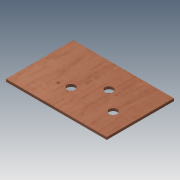
# Autodesk Inventor part: gabarito-porta-cabos
Saved by Autodesk Inventor 2017 (Build 210142000, 142)
## iProperties
Created: 2018-08-29
Part Number: gabarito-porta-cabos
Material: Wood (Oak)
Document SubType Name: Sheet Metal
Designer: Luiz Gustavo
Density: 0.76 g/cm^3
Sheet Metal Rule: Default_mm
Appearance: White Oak - Natural Medium Gloss
Author: Luiz Gustavo
Autodesk Inventor part; units mm, degrees
ref_plane "YZ Plane" through (0, 0, 0) normal (1, 0, 0) x (0, 1, 0)
ref_plane "XZ Plane" through (0, 0, 0) normal (0, 1, 0) x (-1, 0, 0)
ref_plane "XY Plane" through (0, 0, 0) normal (0, 0, 1) x (1, 0, 0)
sketch "Sketch1" plane through (0, 0, 0) normal (0, 0, 1) x (1, 0, 0)
  line L0 (-19.5625, -111.2599) -> (-19.5625, 1344.9999)
  line L1 (40.4374, -111.2599) -> (40.4374, 1344.9999)
  line L2 (14.1874, 432.5) -> (19.1874, 432.5)
  line L3 (19.1874, 427.5) -> (14.1874, 427.5)
  line L4 (26.6874, 422.5) -> (31.6874, 422.5)
  line L5 (31.6874, 417.5) -> (26.6874, 417.5)
  line L6 (1.6874, 422.5) -> (6.6874, 422.5)
  line L7 (6.6874, 417.5) -> (1.6874, 417.5)
  line L8 (4.1874, 417.5) -> (4.1874, 422.5) construction
  line L9 (16.6874, 427.5) -> (16.6874, 432.5) construction
  line L10 (29.1874, 417.5) -> (29.1874, 422.5) construction
  circle A0 centre (4.1874, 420) radius 2.5
  circle A1 centre (16.6874, 430) radius 2.5
  circle A2 centre (29.1874, 420) radius 2.5
  line L11 (40.4374, 405) -> (-19.5625, 405)
  line L12 (-19.5625, 405) -> (-19.5625, 445)
  line L13 (-19.5625, 445) -> (40.4374, 445)
  line L14 (40.4374, 445) -> (40.4374, 405)
  point P0 (0, 0)
  dimension "d0" = 15
  dimension "d1" = 15
  measures "d0" distance from line of L13 A1.centre
  measures "d1" distance from line of point (29.187, 420) L11
extrude "Plate1" add sketch "Sketch1" along normal blind 1.5
equation "\"BendRadius\" = Thickness"
equation "\"BendReliefWidth\" = Thickness"
equation "\"BendReliefDepth\" = 0.5 * Thickness"
equation "\"CornerReliefSize\" = 4 * Thickness"
equation "\"MinimumRemnant\" = 2 * Thickness"
equation "\"TransitionRadius\" = BendRadius"
equation "\"JacobiRadiusSize\" = BendRadius"
equation "\"GapSize\" = Thickness"
equation "\"d2\" = BendRadius"
equation "\"Thickness\" = 1.5"
body "Solid1"
